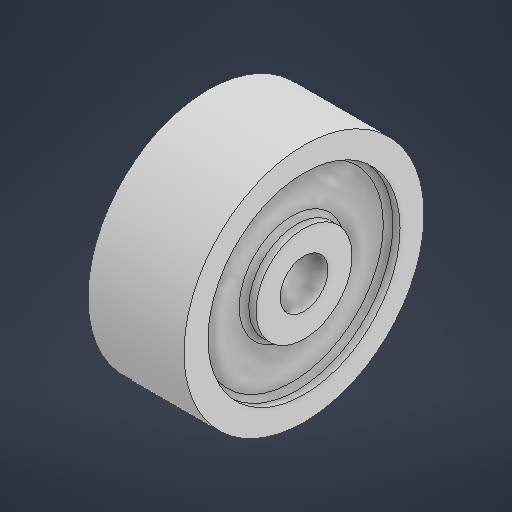
# Autodesk Inventor part: Part1dia14demaio
Saved by Autodesk Inventor 2026 (Build 300175050, 175E)
## iProperties
Created: 2026-05-14
Part Number: Part1dia14demaio
Material: Generic
Document SubType Name: Modeling
Designer: Administrator
Density: 1 g/cm^3
Appearance: Default
Author: Administrator
Autodesk Inventor part; units mm, degrees
ref_plane "YZ Plane" through (0, 0, 0) normal (1, 0, 0) x (0, 1, 0)
ref_plane "XZ Plane" through (0, 0, 0) normal (0, 1, 0) x (-1, 0, 0)
ref_plane "XY Plane" through (0, 0, 0) normal (0, 0, 1) x (1, 0, 0)
sketch "Sketch1" plane through (0, 0, 0) normal (1, 0, 0) x (0, 1, 0)
  circle A0 centre (0, 0) radius 10
  circle A1 centre (0, 0) radius 20
  circle A2 centre (0, 0) radius 40
  circle A3 centre (0, 0) radius 50
  dimension "d0" = 20
  dimension "d1" = 40
  dimension "d2" = 80
  dimension "d3" = 100
  constraints: 4 centre point, 4 coincident
  measures "d0" diameter of A0
  measures "d1" diameter of A1
  measures "d2" diameter of A2
  measures "d3" diameter of A3
extrude "Extrusion1" add sketch "Sketch1" along normal mid plane 40
extrude "Extrusion2" add sketch "Sketch1" along normal mid plane 30 contours A2
fillet "Fillet1" radius 2 1 edges at (15, -40, 0)
fillet "Fillet2" radius 2 1 edges at (15, -20, 0)
fillet "Fillet3" radius 2 1 edges at (-15, -20, 0)
fillet "Fillet4" radius 2 1 edges at (-15, -40, 0)
body "Solid1"
